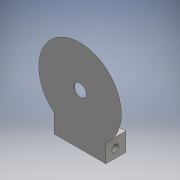
# Autodesk Inventor part: cup
Saved by Autodesk Inventor 2016 (Build 200138000, 138)
## iProperties
Created: 2016-05-03
Part Number: cup
Material: Generic
Document SubType Name: Modeling
Designer: mkepler
Density: 1 g/cm^3
Appearance: Default
Author: mkepler
Autodesk Inventor part; units mm, degrees
ref_plane "YZ Plane" through (0, 0, 0) normal (1, 0, 0) x (0, 1, 0)
ref_plane "XZ Plane" through (0, 0, 0) normal (0, 1, 0) x (-1, 0, 0)
ref_plane "XY Plane" through (0, 0, 0) normal (0, 0, 1) x (1, 0, 0)
sketch "Sketch1" plane through (0, 0, 0) normal (0, 0, 1) x (1, 0, 0)
  line L0 (0, 0) -> (22, 0)
  line L1 (22, 0) -> (22, 2)
  line L2 (22, 0) -> (27, 0)
  line L3 (27, 0) -> (22, 2)
  line L4 (0, 0) -> (0, 3)
  dimension "d0" = 22
  dimension "d1" = 2
  dimension "d2" = 5
  constraints: 10 end point, 2 horizontal, 1 perpendicular, 1 vertical
  measures "d0" distance of L0.start L0.end
  measures "d1" distance of L0.end L1.end
  measures "d2" distance of L0.end L2.end
revolve "Revolution1" add sketch "Sketch1" angle 360 about axis through (0, 0, 0) along (0, 1, 0)
sketch "Sketch2" plane through (0, 0, 0) normal (0, -1, 0) x (1, 0, 0)
  circle A0 centre (0, 0) radius 22
  constraints: 1 centre point, 1 coincident
extrude "Extrusion1" add sketch "Sketch2" against normal blind 0.5
sketch "Sketch3" plane through (0, 0.5, 0) normal (0, 1, 0) x (1, 0, 0)
  circle A0 centre (0, 0) radius 4
  dimension "d6" = 8
  constraints: 1 centre point, 1 coincident
  measures "d6" diameter of A0
extrude "Extrusion2" cut sketch "Sketch3" against normal blind 0.5
sketch "Sketch4" plane through (0, 0, 0) normal (0, -1, 0) x (1, 0, 0)
  circle A0 centre (0, 0) radius 27 projected
  line L0 (-16.875, -28.0969) -> (-16.875, -21.0769)
  line L1 (16.875, -28.0969) -> (16.875, -21.0769)
  circle A1 centre (0, 0) radius 4 projected
  arc A2 (-16.875, -21.0769) -> (16.875, -21.0769) centre (0, 0) ccw
  line L2 (16.875, -28.0969) -> (16.875, -33.0969)
  line L3 (16.875, -33.0969) -> (-16.875, -33.0969)
  line L4 (-16.875, -33.0969) -> (-16.875, -28.0969)
  constraints: 10 end point, 4 point on circle, 1 centre point, 1 coincident, 1 collinear, 1 concentric, 1 perpendicular, 1 vertical
extrude "Extrusion3" add sketch "Sketch4" against normal blind 3 contours A0 L1 L2 L3 L4 L0
sketch "Sketch5" plane through (0, 3, 0) normal (0, 1, 0) x (1, 0, 0)
  arc A0 (16.875, 21.0769) -> (-16.875, 21.0769) centre (0, 0) ccw projected
  circle A1 centre (0, 0) radius 4 projected
  arc A2 (16.875, 21.0769) -> (-16.875, 21.0769) centre (0, 0) ccw
  line L0 (16.875, 21.0769) -> (0, 22)
  circle A3 centre (0, 0) radius 22 projected
  line L1 (-16.875, 21.0769) -> (0, 22)
  constraints: 4 end point, 2 point on circle, 1 centre point, 1 coincident, 1 concentric, 1 vertical alignment, 1 other
extrude "Extrusion4" add sketch "Sketch5" against normal up to next contours L0 A3 L1 A0 | L0 A3 | A3 L1
sketch "Sketch6" plane through (0, 3, 0) normal (0, 1, 0) x (1, 0, 0)
  arc A0 (10, 19.5959) -> (-10, 19.5959) centre (0, 0) ccw
  line L0 (0, 24.98) -> (10, 24.98)
  line L1 (0, 24.98) -> (-10, 24.98)
  line L2 (10, 24.98) -> (10, 19.5959)
  circle A1 centre (0, 0) radius 22 projected
  line L3 (-10, 24.98) -> (-10, 19.5959)
  constraints: 8 end point, 2 point on circle, 1 centre point, 1 coincident, 1 vertical, 2 other
extrude "Extrusion5" add sketch "Sketch6" against normal up to next contours A0 L3 L1 L0 L2
sketch "Sketch7" plane through (0, 3, 0) normal (0, 1, 0) x (1, 0, 0)
  line L0 (16.875, 33.0969) -> (-16.875, 33.0969) projected
  line L1 (-16.875, 33.0969) -> (16.875, 33.0969)
  line L2 (16.875, 21.0769) -> (16.875, 33.0969) projected
  line L3 (16.875, 33.0969) -> (16.875, 21.0769)
  line L4 (10, 21.453) -> (10, 19.5959) projected
  line L5 (10, 21.0769) -> (10, 19.5959)
  line L6 (-16.875, 33.0969) -> (-16.875, 21.0769) projected
  line L7 (-16.875, 33.0969) -> (-16.875, 21.0769)
  line L8 (-10, 21.0769) -> (-10, 19.5959)
  circle A0 centre (0, 0) radius 22 projected
  arc A1 (10, 19.5959) -> (-10, 19.5959) centre (0, 0) ccw
  line L9 (16.875, 21.0769) -> (10, 21.453)
  arc A2 (-16.875, 21.0769) -> (16.875, 21.0769) centre (0, 0) ccw projected
  line L10 (-10, 19.5959) -> (-10, 21.453) projected
  line L11 (-10, 21.453) -> (-10, 19.5959)
  line L12 (-16.875, 21.0769) -> (-10, 21.453) projected
  line L13 (-10, 21.453) -> (-16.875, 21.0769)
  constraints: 16 end point, 3 collinear, 3 point on circle, 1 centre point, 1 coincident, 1 concentric, 1 horizontal, 1 perpendicular, 1 vertical
extrude "Extrusion6" add sketch "Sketch7" along normal blind 10 contours L2 L9 L4 A0 L8 L10 L12 L6 L0
sketch "Sketch9" plane through (-16.875, 0, -33.0969) normal (-1, 0, 0) x (0, 0, 1)
  circle A0 centre (6, 6) radius 2.175
  line L0 (12.02, 0) -> (0, 0) projected
  line L1 (0, 0) -> (0, 13) projected
  point P0 (33.0969, 0)
  dimension "d23" = 4.35
  dimension "d24" = 6
  dimension "d25" = 6
  constraints: 1 centre point
  measures "d23" diameter of A0
  measures "d24" distance from line of L0 A0.centre
  measures "d25" distance from line of L1 A0.centre
hole "Hole1" at (-16.875, 6, -27.0969) direction (1, 0, 0) diameter 4.35 end through all
body "Solid1"
